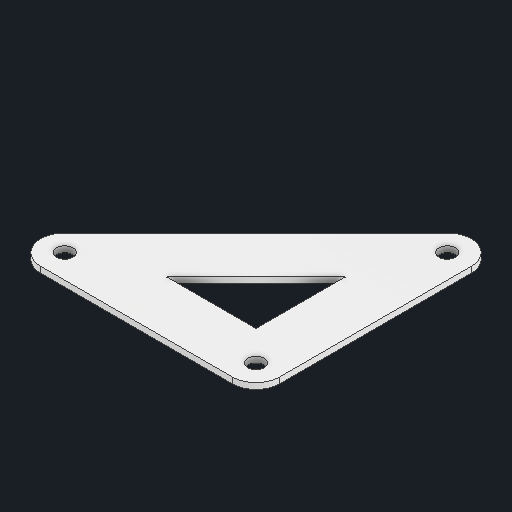
# Autodesk Inventor part: Triangle Gusset
Saved by Autodesk Inventor 2025 (Build 290162000, 162)
## iProperties
Created: 2024-12-30
Part Number: Triangle Gusset
Material: Acetal Resin, White
Document SubType Name: Modeling
Designer: Averey Ku
Density: 1.425 g/cm^3
Appearance: Smooth - White
Author: Averey Ku
Autodesk Inventor part; units mm, degrees
ref_plane "YZ Plane" through (0, 0, 0) normal (1, 0, 0) x (0, 1, 0)
ref_plane "XZ Plane" through (0, 0, 0) normal (0, 1, 0) x (-1, 0, 0)
ref_plane "XY Plane" through (0, 0, 0) normal (0, 0, 1) x (1, 0, 0)
sketch "main" plane through (0, 0, 0) normal (0, 0, 1) x (1, 0, 0)
  circle A0 centre (-24.2926, 27.4457) radius 2.1844
  circle A1 centre (-24.2926, -23.3543) radius 2.1844
  circle A2 centre (26.5074, 27.4457) radius 2.1844
  arc A3 (-30.6426, -23.3543) -> (-19.8025, -27.8444) centre (-24.2926, -23.3543) ccw
  arc A4 (30.9975, 22.9556) -> (26.5074, 33.7957) centre (26.5074, 27.4457) ccw
  arc A5 (-24.2926, 33.7957) -> (-30.6426, 27.4457) centre (-24.2926, 27.4457) ccw
  line L0 (-30.6426, -23.3543) -> (-30.6426, 27.4457)
  line L1 (-24.2926, 33.7957) -> (26.5074, 33.7957)
  line L2 (30.9975, 22.9556) -> (-19.8025, -27.8444)
  line L3 (-16.3551, -4.1915) -> (7.3446, 19.5082)
  line L4 (7.3446, 19.5082) -> (-16.3551, 19.5082)
  line L5 (-16.3551, 19.5082) -> (-16.3551, -4.1915)
  point P0 (-7.9432, 11.0963)
  dimension "d0" = 12.7
  dimension "d1" = 12.7
  dimension "d2" = 12.7
  dimension "d3" = 14.2875
  measures "d0" diameter of A4
  measures "d1" diameter of A5
  measures "d2" diameter of A3
  measures "d3" distance between parallel lines of L2 L3
sketch "Sketch1" plane through (0, 0, 0) normal (0, 1, 0) x (-1, 0, 0)
  circle A0 centre (0, 0) radius 2.1844
  circle A1 centre (0, -50.8) radius 2.1844
  circle A2 centre (50.8, 0) radius 2.1844
  arc A3 (-6.35, -50.8) -> (4.4901, -55.2901) centre (0, -50.8) ccw
  arc A4 (55.2901, -4.4901) -> (50.8, 6.35) centre (50.8, 0) ccw
  arc A5 (0, 6.35) -> (-6.35, 0) centre (0, 0) ccw
  line L0 (-6.35, -50.8) -> (-6.35, 0)
  line L1 (0, 6.35) -> (50.8, 6.35)
  line L2 (55.2901, -4.4901) -> (4.4901, -55.2901)
  line L3 (7.9375, -31.6372) -> (31.6372, -7.9375)
  line L4 (31.6372, -7.9375) -> (7.9375, -7.9375)
  line L5 (7.9375, -7.9375) -> (7.9375, -31.6372)
  constraints: 1 other
extrude "Extrusion1" add sketch "Sketch1" along normal blind 1.5875
body "Solid1"
